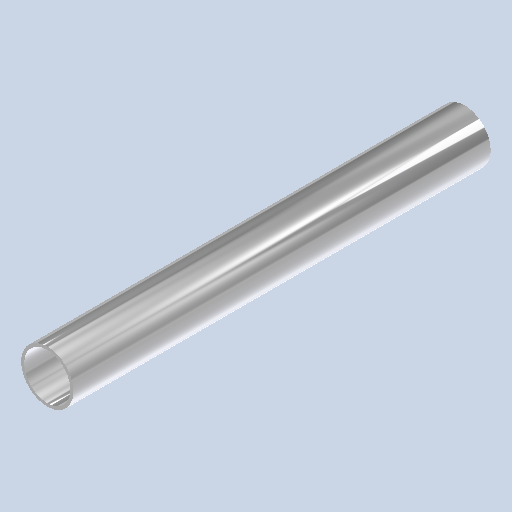
# Autodesk Inventor part: TUBE,AXLE,ARM
Saved by Autodesk Inventor 2025.2 (Build 292293000, 293)
## iProperties
Category: _
Manager: _
ILogicPurgeVersion: 0.0.0.0
OnSaveVersion: 3.5.0.0
OnSaveAssembly: COREAutomationManager
Created: 2025-03-06
Part Number: TUBE,AXLE,ARM
Checked By: 00
Engr Approved By: _
User Status: Work In Process
Material: Aluminum 6061
Description: STANDARD (mm)
Document SubType Name: Modeling
Mfg Approved By: John.Thibert
Designer: John.Thibert
Manufacturer: Standard
Standards Organization: Custom
Mass: 103.164 g
Surface Area: 484.381 cm^2
Volume: 38.2089 cm^3
Density: 2.7 g/cm^3
Appearance: Aluminum - Flat
CN_MASS: 0.1
CN_SERVICEABLE: _
FIRST_DESCRIPTION: _
SECOND_DESCRIPTION: _
THIRD_DESCRIPTION: _
ModelCat: Uncategorized
MaterialName: Aluminum 6061
Subject: _
Author: John.Thibert
Keywords: -
Revision Number: A
Autodesk Inventor part; units mm, degrees
ref_plane "YZ Plane" through (0, 0, 0) normal (1, 0, 0) x (0, 1, 0)
ref_plane "XZ Plane" through (0, 0, 0) normal (0, 1, 0) x (-1, 0, 0)
ref_plane "XY Plane" through (0, 0, 0) normal (0, 0, 1) x (1, 0, 0)
sketch "Sketch2" plane through (0, 0, 0) normal (0, 0, 1) x (1, 0, 0)
  circle A0 centre (0, 0) radius 15.875
  circle A1 centre (0, 0) radius 14.097
  dimension "d0" = 31.75
  dimension "d1" = 1.778
  constraints: 2 centre point, 1 coincident
  measures "d0" diameter of A0
  measures "d1" radial gap between concentric circles of A0 A1
extrude "Extrusion1" add sketch "Sketch2" along normal mid plane 254
body "Solid1"
